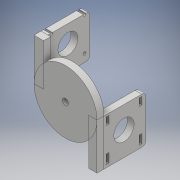
# Autodesk Inventor part: forearm_base
Saved by Autodesk Inventor 2017 (Build 210142000, 142)
## iProperties
Created: 2017-01-01
Part Number: forearm_base
Material: Generic
Document SubType Name: Modeling
Designer: Samanth
Density: 1 g/cm^3
Appearance: Default
Author: Samanth
Autodesk Inventor part; units mm, degrees
ref_plane "YZ Plane" through (0, 0, 0) normal (1, 0, 0) x (0, 1, 0)
ref_plane "XZ Plane" through (0, 0, 0) normal (0, 1, 0) x (-1, 0, 0)
ref_plane "XY Plane" through (0, 0, 0) normal (0, 0, 1) x (1, 0, 0)
sketch "Sketch1" plane through (0, 0, 0) normal (0, 1, 0) x (-1, 0, 0)
  circle A0 centre (0, 0) radius 4.4
  circle A1 centre (0, 0) radius 45
  dimension "d0" = 8.8
  dimension "d1" = 90
  constraints: 2 centre point, 2 coincident
  measures "d0" diameter of A0
  measures "d1" diameter of A1
extrude "Extrusion1" add sketch "Sketch1" along normal mid plane 10
sketch "Sketch2" plane through (0, 5, 0) normal (0, 1, 0) x (1, 0, 0)
  circle A0 centre (0, 0) radius 45 projected
  line L0 (-45, 0) -> (-53, 0)
  line L1 (-53, 0) -> (-53, 49.2006)
  line L2 (45, 0) -> (53, 0)
  line L3 (53, 0) -> (53, 50.9351)
  line L4 (53, 50.9351) -> (45, 50.9351)
  line L5 (45, 50.9351) -> (45, -52.3215)
  line L6 (45, -52.3215) -> (53, -52.3215)
  line L7 (53, -52.3215) -> (53, 50.9351)
  line L8 (-53, 50.9351) -> (-45, 50.9351)
  line L9 (-45, 50.9351) -> (-45, -59.1596)
  line L10 (-45, -59.1596) -> (-53, -59.1596)
  line L11 (-53, -59.1596) -> (-53, 50.9351)
  line L12 (-45, 0) -> (-31.2804, 0)
  line L13 (-31.2804, 0) -> (-31.2804, -60.0944)
  line L14 (-31.2804, -60.0944) -> (-45, -60.0944)
  line L15 (-45, -60.0944) -> (-45, 0)
  line L16 (45, 0) -> (33.3273, 0)
  line L17 (33.3273, 0) -> (33.3273, 65.7607)
  line L18 (33.3273, 65.7607) -> (45, 65.7607)
  line L19 (45, 65.7607) -> (45, 0)
  line L20 (-31.2804, 0) -> (-43.8048, 0)
  line L21 (-43.8048, 0) -> (-43.8048, -65.7457)
  line L22 (-43.8048, -65.7457) -> (-31.2804, -65.7457)
  line L23 (-31.2804, -65.7457) -> (-31.2804, 0)
  dimension "d4" = 8
  dimension "d5" = 8
  constraints: 48 end point, 10 parallel, 7 horizontal, 7 perpendicular, 2 point on circle, 1 point on line
  measures "d4" distance of L0.start L0.end
  measures "d5" distance of L2.start L2.end
extrude "Extrusion2" add sketch "Sketch2" along normal blind 60 contours L16 L17 A0 | A0 L17 L18 L19 L5 | L13 L14 L21 A0 | A0 L21 L12 L13 | L12 L21 A0 | A0 L21 L14 L15 L9
sketch "Sketch3" plane through (0, 5, 0) normal (0, 1, 0) x (1, 0, 0)
  point P0 (0, 0)
sketch "Sketch4" plane through (-31.2804, 5, 60.0944) normal (1, 0, 0) x (0, 0, -1)
  line L0 (0, 0) -> (27.7442, 0) projected
  line L1 (0, 0) -> (0, 57)
  line L2 (0, 0) -> (0, 60) projected
  line L3 (60.0944, 0) -> (60.0944, 60) projected
  line L4 (60.0944, 0) -> (15.0944, 0) projected
  circle A0 centre (25.0348, 28.5) radius 14.25
  line L5 (1.4498, 4.93) -> (48.6198, 4.93)
  line L6 (1.4498, 4.93) -> (48.6198, 52.07) construction
  line L7 (48.6198, 4.93) -> (1.4498, 52.07) construction
  circle A1 centre (48.6198, 52.07) radius 2
  circle A2 centre (48.6198, 4.93) radius 2
  circle A3 centre (1.4498, 4.93) radius 2
  circle A4 centre (1.4498, 52.07) radius 2
  circle A5 centre (91.5944, 28.5) radius 14.5222
  line L8 (68.0094, 4.93) -> (115.1794, 52.07) construction
  line L9 (115.1794, 4.93) -> (68.0094, 52.07) construction
  line L10 (62.8112, 54.07) -> (73.2076, 54.07)
  line L11 (73.2076, 54.07) -> (73.2076, 50.07)
  line L12 (73.2076, 50.07) -> (62.8112, 50.07)
  line L13 (62.8112, 50.07) -> (62.8112, 54.07)
  line L14 (62.8112, 54.07) -> (73.2076, 50.07) construction
  line L15 (73.2076, 54.07) -> (62.8112, 50.07) construction
  line L16 (62.8112, 6.93) -> (73.2076, 6.93)
  line L17 (73.2076, 6.93) -> (73.2076, 2.93)
  line L18 (73.2076, 2.93) -> (62.8112, 2.93)
  line L19 (62.8112, 2.93) -> (62.8112, 6.93)
  line L20 (66.1428, 5.6482) -> (73.2076, 2.93) construction
  line L21 (73.2076, 6.93) -> (62.8112, 2.93) construction
  line L22 (121.5703, 54.07) -> (108.7885, 54.07)
  line L23 (108.7885, 54.07) -> (108.7885, 50.07)
  line L24 (108.7885, 50.07) -> (121.5703, 50.07)
  line L25 (121.5703, 50.07) -> (121.5703, 54.07)
  line L26 (121.5703, 54.07) -> (108.7885, 50.07) construction
  line L27 (108.7885, 54.07) -> (121.5703, 50.07) construction
  line L28 (121.5703, 6.93) -> (108.7885, 6.93)
  line L29 (108.7885, 6.93) -> (108.7885, 2.93)
  line L30 (108.7885, 2.93) -> (121.5703, 2.93)
  line L31 (121.5703, 2.93) -> (121.5703, 6.93)
  line L32 (121.5703, 6.93) -> (108.7885, 2.93) construction
  line L33 (108.7885, 6.93) -> (121.5703, 2.93) construction
  point P0 (60.0944, -5)
  dimension "d8" = 57
  dimension "d13" = 4
  dimension "d14" = 4
  constraints: 60 end point, 8 parallel, 6 centre point, 5 horizontal, 5 point on line, 4 coincident, 4 midpoint, 4 perpendicular
  measures "d8" distance of L0.start L1.end
  measures "d13" diameter of A2
  measures "d14" diameter of A3
extrude "Extrusion3" cut sketch "Sketch4" along normal mid plane 660
sketch "Sketch5" plane through (33.3273, 5, -65.7607) normal (-1, 0, 0) x (0, 0, 1)
  point P0 (65.7607, -5)
sketch "Sketch6" plane through (0, -5, 0) normal (0, -1, 0) x (1, 0, 0)
  line L0 (45, 0) -> (45, -65.7607) projected
  line L1 (33.3273, 0) -> (45, 0) projected
  line L2 (45, -65.7607) -> (33.3273, -65.7607)
  line L3 (33.3273, -65.7607) -> (33.3273, 0)
  line L4 (33.3273, 0) -> (45, 0)
  line L5 (45, 0) -> (45, -65.7607)
  circle A0 centre (0, 0) radius 45 projected
  line L6 (-31.2804, 60.0944) -> (-45, 60.0944) projected
  line L7 (-45, 0) -> (-31.2804, 0)
  line L8 (-31.2804, 0) -> (-31.2804, 60.0944)
  line L9 (-31.2804, 60.0944) -> (-45, 60.0944)
  line L10 (-45, 60.0944) -> (-45, 0)
  constraints: 16 end point, 4 parallel, 2 horizontal, 2 perpendicular, 1 point on circle, 1 point on line
extrude "Extrusion4" add sketch "Sketch6" against normal blind 10 separate body contours A0 L3 L1 | L0 L2 L3 A0 | L8 L7 A0 | A0 L10 L6 L8
fillet "Fillet1" radius 6 4 edges at (-38.1402, 65, 0) (-38.1402, 65, 60.0944) (39.1636, 65, 0) (39.1636, 65, -65.7607)
sketch "Sketch7" plane through (0, 65, 0) normal (0, 1, 0) x (1, 0, 0)
  line L0 (-31.2804, 0) -> (-45, 0) projected
  line L1 (-31.2804, -60.0944) -> (-31.2804, -32.3502) projected
  line L2 (-35.091, 0) -> (-31.2804, 0)
  line L3 (-31.2804, 0) -> (-31.2804, -60.0944)
  line L4 (-31.2804, -60.0944) -> (-35.091, -60.0944)
  line L5 (-35.091, -60.0944) -> (-35.091, 0)
  line L6 (45, 0) -> (33.3273, 0) projected
  line L7 (45, 65.7607) -> (33.3273, 65.7607) projected
  line L8 (33.3273, 0) -> (35.4604, 0)
  line L9 (35.4604, 0) -> (35.4604, 65.7607)
  line L10 (35.4604, 65.7607) -> (33.3273, 65.7607)
  line L11 (33.3273, 65.7607) -> (33.3273, 0)
  point P0 (0, 0)
  constraints: 16 end point, 4 parallel, 2 horizontal, 2 perpendicular, 2 point on line
extrude "Extrusion5" cut sketch "Sketch7" against normal blind 60 bodies 1 2
body "Solid1"
body "Solid2"
